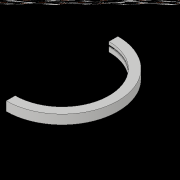
# Autodesk Inventor part: Outer_Shell
Saved by Autodesk Inventor 2017 (Build 210142000, 142)
## iProperties
Created: 2017-01-10
Part Number: Outer_Shell
Material: Generic
Document SubType Name: Modeling
Designer: David Kopala
Density: 1 g/cm^3
Appearance: Default
Author: David Kopala
Autodesk Inventor part; units mm, degrees
ref_plane "YZ Plane" through (0, 0, 0) normal (1, 0, 0) x (0, 1, 0)
ref_plane "XZ Plane" through (0, 0, 0) normal (0, 1, 0) x (-1, 0, 0)
ref_plane "XY Plane" through (0, 0, 0) normal (0, 0, 1) x (1, 0, 0)
sketch "Sketch1" plane through (0, 0, 0) normal (1, 0, 0) x (0, 1, 0)
  line L0 (0, 0) -> (50.8, 0)
  line L1 (0, 266.7) -> (0, 317.5)
  line L2 (0, 317.5) -> (52.3875, 317.5)
  line L3 (52.3875, 317.5) -> (52.3875, 266.7)
  line L4 (49.2125, 314.325) -> (3.175, 314.325)
  line L5 (3.175, 314.325) -> (3.175, 269.875)
  line L6 (49.2125, 269.875) -> (49.2125, 314.325)
  line L7 (26.8351, 281.7194) -> (26.8351, 253.7977)
  line L8 (35.7251, 282.3166) -> (35.7251, 256.0374)
  line L9 (0, 266.7) -> (26.8351, 266.7)
  line L10 (35.7251, 266.7) -> (52.3875, 266.7)
  line L11 (3.175, 269.875) -> (26.8351, 269.875)
  line L12 (35.7251, 269.875) -> (49.2125, 269.875)
  point P0 (3.175, 314.325)
  dimension "d0" = 50.8
  dimension "d1" = 52.3875
  dimension "d3" = 50.8
  dimension "d4" = 52.3875
  dimension "d5" = 3.175
  dimension "d6" = 3.175
  dimension "d7" = 3.175
  dimension "d8" = 3.175
  dimension "d9" = 3.175
  dimension "d11" = 3.175
  dimension "d13" = 23.6601
  dimension "d14" = 8.89
  constraints: 26 end point, 4 horizontal, 4 point on line, 3 parallel, 3 vertical, 2 perpendicular
  measures "d0" distance of L0.start L0.end
  measures "d1" distance of L1.start L3.end
  measures "d3" distance of L1.start L1.end
  measures "d4" distance of L1.end L2.end
  measures "d5" distance from line of L3 L4.start
  measures "d6" distance from line of L2 L4.start
  measures "d7" distance from line of L2 point (3.175, 314.325)
  measures "d8" distance from line of L1 point (3.175, 314.325)
  measures "d9" distance from line of L1 L5.end
  measures "d11" distance from line of L3 point (49.213, 269.875)
  measures "d13" distance between parallel lines of L5 L7
  measures "d14" distance between parallel lines of L7 L8
revolve "Revolution1" add sketch "Sketch1" angle 180 about axis through (0, 0, 0) along (0, 1, 0)
body "Solid1"
